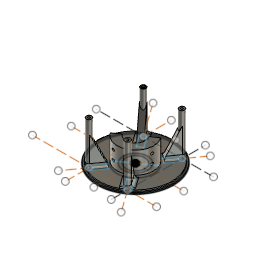
sphere_PS2 v9 (Autodesk Fusion 360 design; units mm, degrees)
Autodesk Fusion 360 part; units mm, degrees
sketch "Skizze1" plane through (0, 0, 0) normal (0, 0, 1) x (1, 0, 0)
  circle A0 centre (0, 0) radius 62.5
  circle A1 centre (0, 0) radius 59.85
  circle A2 centre (0, 0) radius 20
  circle A3 centre (0, 0) radius 15.65
  circle A4 centre (0, 0) radius 6.2
  arc A5 (-24.4487, -17.3857) -> (24.4487, 17.3857) centre (0, 0) ccw
  circle A6 centre (0, 0) radius 2
  line L0 (0, -68.8884) -> (0, 67.0107) construction
  line L1 (80, -45) -> (-125.6154, -45) construction
  line L2 (84.256, 45) -> (-110, 45) construction
  line L3 (32, -72.1137) -> (32, 83.7416) construction
  line L4 (-32, -84.1555) -> (-32, 91.3107) construction
  line L5 (58.3516, -82.0569) -> (-71.7084, 100.84) construction
  line L6 (51.4969, 72.4176) -> (-53.0644, -74.6218) construction
  line L7 (28.3327, -47.6079) -> (15.5832, -29.6788)
  line L8 (35.6673, -42.3921) -> (22.9178, -24.4631)
  line L9 (-28.3327, -47.6079) -> (-15.5832, -29.6788)
  line L10 (-35.6673, -42.3921) -> (-22.9178, -24.4631)
  line L11 (-35.6673, 42.3921) -> (-22.9178, 24.4631)
  line L12 (-28.3327, 47.6079) -> (-15.5832, 29.6788)
  line L13 (28.3327, 47.6079) -> (15.5832, 29.6788)
  line L14 (35.6673, 42.3921) -> (22.9178, 24.4631)
  line L15 (22.9178, -24.4631) -> (15.5832, -29.6788)
  arc A7 (28.3327, -47.6079) -> (35.6673, -42.3921) centre (32, -45) ccw
  line L16 (-15.5832, -29.6788) -> (-22.9178, -24.4631)
  arc A8 (-35.6673, -42.3921) -> (-28.3327, -47.6079) centre (-32, -45) ccw
  line L17 (-15.5832, 29.6788) -> (-22.9178, 24.4631)
  arc A9 (-28.3327, 47.6079) -> (-35.6673, 42.3921) centre (-32, 45) ccw
  line L18 (22.9178, 24.4631) -> (15.5832, 29.6788)
  arc A10 (35.6673, 42.3921) -> (28.3327, 47.6079) centre (32, 45) ccw
  circle A11 centre (32, 45) radius 4.5
  circle A12 centre (-32, 45) radius 4.5
  circle A13 centre (-32, -45) radius 4.5
  circle A14 centre (32, -45) radius 4.5
  line L19 (24.4487, 17.3857) -> (-24.4487, -17.3857)
  line L20 (80, 0) -> (-106.3472, 0) construction
  circle A15 centre (-32, 45) radius 3
  dimension "d1" = 125
  dimension "d2" = 119.7
  dimension "d3" = 40
  dimension "d4" = 31.3
  dimension "d5" = 12.4
  dimension "d6" = 30
  dimension "d15" = 4
  dimension "d54" = 45
  dimension "d55" = 45
  dimension "d56" = 32
  dimension "d57" = 32
  dimension "d66" = 9
  dimension "d67" = 9
  dimension "d68" = 9
  dimension "d69" = 9
  dimension "d100" = 6
  constraint coincident A0.centre A1.centre
  constraint concentric A0 A1
  constraint concentric A3 A6
  constraint vertical L0
  constraint horizontal L2
  constraint vertical L3
  constraint perpendicular L1 L4
  constraint coincident A0.centre L6
  constraint coincident A0.centre L5
  constraint parallel L6 L14
  constraint parallel L6 L13
  constraint parallel L5 L12
  constraint parallel L5 L11
  constraint parallel L6 L10
  constraint parallel L6 L9
  constraint parallel L5 L7
  constraint parallel L5 L8
  constraint perpendicular L5 L15
  constraint coincident L8 L15.start
  constraint coincident L8.end L15.start
  constraint coincident L7 L15.end
  constraint coincident L7.end L15
  constraint coincident L3 A7.centre
  constraint coincident L1 A7.centre
  constraint perpendicular L6 L16
  constraint coincident L10 L16.end
  constraint coincident L9 L16.start
  constraint coincident L9.end L16
  constraint coincident L10.end L16
  constraint coincident L1 A8.centre
  constraint coincident L6 A8.centre
  constraint perpendicular L5 L17
  constraint coincident L11.end L17
  constraint coincident L12 L17.start
  constraint coincident L11 L17.end
  constraint coincident L12.end L17
  constraint coincident L5 A9.centre
  constraint coincident L2 A9.centre
  constraint perpendicular L6 L18
  constraint coincident L13 L18.end
  constraint coincident L14 L18.start
  constraint coincident L14.end L18
  constraint coincident L13.end L18
  constraint coincident L6 A10.centre
  constraint coincident L2 A10.centre
  constraint concentric A10 A11
  constraint concentric A9 A12
  constraint concentric A8 A13
  constraint concentric A7 A14
  constraint coincident A0.centre L19
  constraint horizontal L20
  constraint perpendicular L5 L19
  constraint coincident A5.end L19
  constraint coincident A5.start L19
  constraint coincident A5 L19.end
  constraint coincident A5 L19.start
  constraint concentric A9 A15
  measures "d1" diameter of A0
  measures "d2" diameter of A1
  measures "d3" diameter of A2
  measures "d4" diameter of A3
  measures "d5" diameter of A4
  measures "d6" radius of A5
  measures "d15" diameter of A6
  measures "d54" distance of A0.centre L2
  measures "d55" distance of A0.centre L1
  measures "d56" distance of A0.centre L4
  measures "d57" distance of A0.centre L3
  measures "d66" diameter of A11
  measures "d67" diameter of A12
  measures "d68" diameter of A13
  measures "d69" diameter of A14
  measures "d100" diameter of A15
extrude "Extrusion1" add sketch "Skizze1" along normal blind 2 contours A0 | A1 | A2 A3 L19 | A2 A5 L19 | A2 A3 L19 | A3 A4 L19 | A3 A4 L19 | A4 A6 L19 | A4 A6 L19 | A7 A14 | L7 L8 L15 A14 | L9 L10 L16 A13 | A8 A13 | L11 L12 L17 A12 | A9 A12 | L13 L14 L18 A11 | A10 A11 | A15
extrude "Extrusion2" add sketch "Skizze1" along normal blind 4 contours A1 | A2 A3 L19 | A2 A5 L19 | A2 A3 L19 | A3 A4 L19 | A3 A4 L19 | A7 A14 | L7 L8 L15 A14 | L9 L10 L16 A13 | A8 A13 | L11 L12 L17 A12 | A9 A12 | L13 L14 L18 A11 | A10 A11 | A15
extrude "Extrusion3" add sketch "Skizze1" along normal blind 9 contours A2 A3 L19 | A2 A3 L19
extrude "Extrusion4" add sketch "Skizze1" along normal blind 40 contours A2 A3 L19 | A2 A5 L19 picked at (-14.4863, -11.5112)
extrude "Extrusion10" add sketch "Skizze1" along normal blind 50 contours L7 L8 L15 A14 | L9 L10 L16 A13 | L11 L12 L17 A12 | L13 L14 L18 A11
ref_plane "Arbeitsebene3" through (0, 0, 0) normal (0.814955, -0.579524, 0) x (0.579524, 0.814955, 0)
sketch "Skizze4" plane through (0, 0, 0) normal (0.814955, -0.579524, 0) x (0.579524, 0.814955, 0)
  line L0 (55, 50) -> (33, 50)
  line L1 (-33, 50) -> (-55, 50)
  line L2 (55, 50) -> (33, 4)
  line L3 (73.2312, 4) -> (-81.5781, 4) construction
  line L4 (33, 27.5575) -> (33, -13.6721) construction
  line L5 (-33, 28.7468) -> (-33, -25) construction
  line L6 (55, 50) -> (55, -48.5325) construction
  line L7 (-55, 50) -> (-55, -41.8091) construction
  line L8 (-55, 50) -> (-33, 4)
  line L9 (-33, 4) -> (-33, 50)
  line L10 (33, 4) -> (33, 50)
  point P0 (33, 4)
  point P1 (-33, 4)
  dimension "d72" = 50
  dimension "d73" = 50
  dimension "d75" = 4
  dimension "d76" = 33
  dimension "d77" = 33
  dimension "d78" = 55
  dimension "d79" = 55
  constraint horizontal L0
  constraint horizontal L1
  constraint horizontal L3
  constraint perpendicular L3 L4
  constraint vertical L5
  constraint coincident L4 P0
  constraint coincident L3 P0
  constraint coincident L5 P1
  constraint coincident L3 P1
  constraint coincident L2 P0
  constraint vertical L6
  constraint vertical L7
  constraint coincident L0 L2.start
  constraint coincident L1 L7.start
  constraint coincident L1.end L7
  constraint coincident L0.start L6
  constraint coincident L2 L0.start
  constraint coincident P0 L2.end
  constraint coincident L0.start L2.start
  constraint coincident L1.end L7.start
  constraint coincident P1 L8.end
  constraint coincident L1 L9.end
  constraint perpendicular L1 L9
  constraint coincident L0 L10.end
  constraint perpendicular L0 L10
  constraint coincident L0.end L10
  constraint coincident L1.start L5
  measures "d72" distance of L1 origin
  measures "d73" distance of L0 origin
  measures "d75" distance of L3 origin
  measures "d76" distance of L4 origin
  measures "d77" distance of origin L5
  measures "d78" distance of origin L7
  measures "d79" distance of L6 origin
extrude "Extrusion11" cut sketch "Skizze4" along normal mid plane 20
ref_plane "Arbeitsebene4" through (0, 0, 0) normal (-0.814955, -0.579524, 0) x (0.579524, -0.814955, 0)
sketch "Skizze5" plane through (0, 0, 0) normal (-0.814955, -0.579524, 0) x (0.579524, -0.814955, 0)
  line L0 (-55, 50) -> (-33, 50)
  line L1 (4.8827, 50) -> (55, 50)
  line L2 (-55, 70) -> (-55, -33.6954) construction
  line L3 (55, 69.2155) -> (55, -50) construction
  line L4 (-103.884, 4) -> (120, 4) construction
  line L5 (-33, 50) -> (-33, 4)
  line L6 (33, 50) -> (33, 4)
  line L7 (-55, 50) -> (-33, 4)
  line L8 (55, 50) -> (33, 4)
  dimension "d87" = 50
  dimension "d88" = 50
  dimension "d89" = 55
  dimension "d90" = 55
  dimension "d91" = 4
  dimension "d94" = 22
  dimension "d95" = 22
  constraint horizontal L0
  constraint horizontal L1
  constraint vertical L2
  constraint vertical L3
  constraint horizontal L4
  constraint vertical L5
  constraint perpendicular L4 L6
  constraint coincident L1 L6.start
  constraint coincident L0.end L5
  constraint coincident L0 L5.start
  constraint coincident L4 L5.end
  constraint coincident L4 L6.end
  constraint coincident L1.end L3
  constraint coincident L0.start L2
  constraint coincident L5.end L7.end
  constraint coincident L0.start L7.start
  constraint coincident L6.end L8.end
  constraint coincident L1.end L8.start
  measures "d87" distance of L1 origin
  measures "d88" distance of L0 origin
  measures "d89" distance of origin L2
  measures "d90" distance of origin L3
  measures "d91" distance of origin L4
  measures "d94" distance of L2 L5
  measures "d95" distance of L3 L6
extrude "Extrusion12" cut sketch "Skizze5" along normal mid plane 20
extrude "Extrusion13" add sketch "Skizze1" along normal blind 72 contours A7 A14 | A8 A13 | A10 A11 | A15
extrude "Extrusion14" add sketch "Skizze1" along normal blind 71 contours A9 A12
fillet "Abrundung3" radius 5 3 edges at (-29.2925, 33.4276, 4) (-34.6079, 48.6673, 4) (-21.9579, 38.6433, 4)
fillet "Abrundung4" radius 5 3 edges at (-21.9579, -38.6433, 4) (-34.6079, -48.6673, 4) (-29.2925, -33.4276, 4)
fillet "Abrundung5" radius 5 3 edges at (29.2925, -33.4276, 4) (34.6079, -48.6673, 4) (21.9579, -38.6433, 4)
fillet "Abrundung6" radius 5 3 edges at (21.9579, 38.6433, 4) (34.6079, 48.6673, 4) (29.2925, 33.4276, 4)
ref_plane "Arbeitsebene5" through (-16.2833, -16.4875, 22) normal (-0.579524, 0.814955, 0) x (-0.814955, -0.579524, 0)
sketch "Skizze2" plane through (2.3181, -3.2598, 0) normal (-0.579524, 0.814955, 0) x (0.814955, 0.579524, 0)
  line L0 (23, -47.583) -> (23, 16) construction
  line L1 (-23, -47) -> (-23, 14.5084) construction
  line L2 (39.9606, -30) -> (-42.0458, -30) construction
  line L3 (40.0778, -15) -> (-41.9288, -15) construction
  line L4 (24.6743, -32.9) -> (26.3486, -30)
  line L5 (26.3486, -30) -> (24.6743, -27.1)
  line L6 (24.6743, -27.1) -> (21.3257, -27.1)
  line L7 (21.3257, -27.1) -> (19.6514, -30)
  line L8 (19.6514, -30) -> (21.3257, -32.9)
  line L9 (21.3257, -32.9) -> (24.6743, -32.9)
  line L10 (24.6743, -17.9) -> (26.3486, -15)
  line L11 (26.3486, -15) -> (24.6743, -12.1)
  line L12 (24.6743, -12.1) -> (21.3257, -12.1)
  line L13 (21.3257, -12.1) -> (19.6514, -15)
  line L14 (19.6514, -15) -> (21.3257, -17.9)
  line L15 (21.3257, -17.9) -> (24.6743, -17.9)
  line L16 (-21.3257, -32.9) -> (-19.6514, -30)
  line L17 (-19.6514, -30) -> (-21.3257, -27.1)
  line L18 (-21.3257, -27.1) -> (-24.6743, -27.1)
  line L19 (-24.6743, -27.1) -> (-26.3486, -30)
  line L20 (-26.3486, -30) -> (-24.6743, -32.9)
  line L21 (-24.6743, -32.9) -> (-21.3257, -32.9)
  line L22 (-21.3257, -17.9) -> (-19.6514, -15)
  line L23 (-19.6514, -15) -> (-21.3257, -12.1)
  line L24 (-21.3257, -12.1) -> (-24.6743, -12.1)
  line L25 (-24.6743, -12.1) -> (-26.3486, -15)
  line L26 (-26.3486, -15) -> (-24.6743, -17.9)
  line L27 (-24.6743, -17.9) -> (-21.3257, -17.9)
  line L28 (26.3486, -32.9) -> (19.6514, -32.9)
  line L29 (19.6514, -32.9) -> (19.6514, -30)
  line L30 (19.6514, -30) -> (26.3486, -30)
  line L31 (26.3486, -30) -> (26.3486, -32.9)
  line L32 (-19.6514, -32.9) -> (-26.3486, -32.9)
  line L33 (-26.3486, -32.9) -> (-26.3486, -30)
  line L34 (-26.3486, -30) -> (-19.6514, -30)
  line L35 (-19.6514, -30) -> (-19.6514, -32.9)
  line L36 (-19.6514, -17.9) -> (-26.3486, -17.9)
  line L37 (-26.3486, -17.9) -> (-26.3486, -15)
  line L38 (-26.3486, -15) -> (-19.6514, -15)
  line L39 (-19.6514, -15) -> (-19.6514, -17.9)
  line L40 (26.3486, -17.9) -> (19.6514, -17.9)
  line L41 (19.6514, -17.9) -> (19.6514, -15)
  line L42 (19.6514, -15) -> (26.3486, -15)
  line L43 (26.3486, -15) -> (26.3486, -17.9)
  circle A0 centre (23, -30) radius 1.75
  circle A1 centre (23, -15) radius 1.75
  circle A2 centre (-23, -30) radius 1.75
  circle A3 centre (-23, -15) radius 1.75
  line L44 (-15.65, -9) -> (-20, -9)
  line L45 (-20, -9) -> (-20, -4)
  line L46 (-20, -4) -> (-30, -4)
  line L47 (-30, -4) -> (-30, -40)
  line L48 (-30, -40) -> (-15.65, -40)
  line L49 (-15.65, -40) -> (-15.65, -9)
  line L50 (67, 0) -> (-48, 0) construction
  line L51 (83.9354, 0) -> (-86.4902, 0)
  line L52 (-15.713, 0) -> (74.6088, 0)
  point P0 (23, -30)
  point P1 (23, -15)
  point P2 (-23, -15)
  point P3 (-23, -30)
  point P4 (23, -30)
  point P5 (23, -15)
  point P6 (-23, -30)
  point P7 (-23, -15)
  dimension "d24" = 23
  dimension "d25" = 23
  dimension "d26" = 30
  dimension "d27" = 15
  dimension "d28" = 5.8
  dimension "d29" = 5.8
  dimension "d30" = 5.8
  dimension "d31" = 5.8
  dimension "d32" = 3.5
  dimension "d33" = 3.5
  dimension "d34" = 3.5
  dimension "d35" = 3.5
  constraint vertical L0
  constraint vertical L1
  constraint coincident L2 P4
  constraint coincident L0 P4
  constraint coincident L3 P5
  constraint coincident L0 P5
  constraint coincident L1 P7
  constraint coincident L3 P7
  constraint coincident L1 P6
  constraint coincident L2 P6
  constraint coincident P4 P0
  constraint coincident P5 P1
  constraint coincident P6 P3
  constraint coincident P7 P2
  constraint horizontal L28
  constraint vertical L29
  constraint horizontal L30
  constraint vertical L31
  constraint coincident P4 L30
  constraint coincident L7.end L8.start
  constraint coincident L4.end L5.start
  constraint coincident L8.end L28
  constraint horizontal L32
  constraint vertical L33
  constraint horizontal L34
  constraint vertical L35
  constraint coincident P6 L34
  constraint coincident L19.end L20.start
  constraint coincident L16.end L17.start
  constraint coincident L16.start L32
  constraint horizontal L36
  constraint vertical L37
  constraint horizontal L38
  constraint vertical L39
  constraint coincident P7 L38
  constraint coincident L25.end L26.start
  constraint coincident L26.end L36
  constraint coincident L22.end L23.start
  constraint horizontal L40
  constraint vertical L41
  constraint horizontal L42
  constraint vertical L43
  constraint coincident P5 L42
  constraint coincident L13.end L14.start
  constraint coincident L10.end L11.start
  constraint coincident L14.end L40
  constraint horizontal L50
  constraint coincident L50 origin
  constraint parallel L2 L51
  constraint parallel L3 L52
  measures "d24" distance of L0 origin
  measures "d25" distance of L1 origin
  measures "d26" distance of origin L2
  measures "d27" distance of origin L3
  measures "d28" distance of L6 L9
  measures "d29" distance of L12 L15
  measures "d30" distance of L18 L21
  measures "d31" distance of L24 L27
  measures "d32" diameter of A3
  measures "d33" diameter of A2
  measures "d34" diameter of A0
  measures "d35" diameter of A1
extrude "Extrusion6" cut sketch "Skizze2" along normal mid plane 80 contours L30 A0 | L30 A0 | L42 A1 | L42 A1 | L34 A2 | L34 A2 | L38 A3 | L38 A3
extrude "Extrusion7" cut sketch "Skizze2" along normal mid plane 2.8 contours L4 L8 L9 L28 L30 A0 | L4 L28 L31 | L5 L6 L7 L30 A0 | L8 L28 L29 | L10 L14 L15 L40 L42 A1 | L10 L40 L43 | L11 L12 L13 L42 A1 | L14 L40 L41 | L16 L20 L21 L32 L34 A2 | L16 L32 L35 | L17 L18 L19 L34 A2 | L20 L32 L33 | L22 L26 L27 L36 L38 A3 | L22 L36 L39 | L23 L24 L25 L38 A3 | L26 L36 L37
ref_plane "Arbeitsebene2" through (-32, -45, 66) normal (0, 0, 1) x (1, 0, 0)
sketch "Skizze3" plane through (0, 0, 66) normal (0, 0, 1) x (1, 0, 0)
  line L0 (47.2936, -66.5067) -> (-50.249, 70.6626) construction
  line L1 (-42.6718, -60.0072) -> (38.3749, 53.9647) construction
  line L2 (-31.9062, -41.6527) -> (-34.852, -43.2451)
  line L3 (-34.852, -43.2451) -> (-34.9457, -46.5925)
  line L4 (-34.9457, -46.5925) -> (-32.0938, -48.3473)
  line L5 (-32.0938, -48.3473) -> (-29.148, -46.7549)
  line L6 (-29.148, -46.7549) -> (-29.0543, -43.4075)
  line L7 (-29.0543, -43.4075) -> (-31.9062, -41.6527)
  line L8 (-28.9183, 43.6898) -> (-29.3245, 47.0137)
  line L9 (-29.3245, 47.0137) -> (-32.4061, 48.3239)
  line L10 (-32.4061, 48.3239) -> (-35.0817, 46.3102)
  line L11 (-35.0817, 46.3102) -> (-34.6755, 42.9863)
  line L12 (-34.6755, 42.9863) -> (-31.5939, 41.6761)
  line L13 (-31.5939, 41.6761) -> (-28.9183, 43.6898)
  line L14 (31.9063, 41.6527) -> (34.852, 43.2452)
  line L15 (34.852, 43.2452) -> (34.9457, 46.5925)
  line L16 (34.9457, 46.5925) -> (32.0937, 48.3473)
  line L17 (32.0937, 48.3473) -> (29.148, 46.7548)
  line L18 (29.148, 46.7548) -> (29.0543, 43.4075)
  line L19 (29.0543, 43.4075) -> (31.9063, 41.6527)
  line L20 (35.0817, -46.3102) -> (34.6755, -42.9863)
  line L21 (34.6755, -42.9863) -> (31.5939, -41.6761)
  line L22 (31.5939, -41.6761) -> (28.9183, -43.6898)
  line L23 (28.9183, -43.6898) -> (29.3245, -47.0137)
  line L24 (29.3245, -47.0137) -> (32.4061, -48.3239)
  line L25 (32.4061, -48.3239) -> (35.0817, -46.3102)
  circle A0 centre (-32, 45) radius 1.75
  circle A1 centre (-32, -45) radius 1.75
  circle A2 centre (32, -45) radius 1.75
  circle A3 centre (32, 45) radius 1.75
  line L26 (-32, -63.1927) -> (-32, 71.2003) construction
  line L27 (-86.7098, 45) -> (100, 45) construction
  line L28 (-83.1793, -45) -> (68.6306, -45) construction
  line L29 (32, -70) -> (32, 90) construction
  point P0 (-32, -45)
  point P1 (-32, 45)
  point P2 (32, 45)
  point P3 (32, -45)
  point P4 (-32, -45)
  point P5 (-32, 45)
  point P6 (32, 45)
  point P7 (32, -45)
  point P8 (-32, 45)
  point P9 (102.7985, 45)
  point P10 (-3.6645, -45)
  point P11 (-32, -45)
  point P12 (32, 45)
  point P13 (32, -45)
  dimension "d42" = 5.8
  dimension "d43" = 5.8
  dimension "d44" = 5.8
  dimension "d45" = 5.8
  dimension "d46" = 3.5
  dimension "d47" = 3.5
  dimension "d48" = 3.5
  dimension "d49" = 3.5
  dimension "d113" = 32
  dimension "d114" = 45
  dimension "d115" = 45
  dimension "d116" = 32
  constraint coincident L0 origin
  constraint coincident origin L1
  constraint coincident L1 P11
  constraint coincident L0 P8
  constraint coincident L1 P12
  constraint coincident L0 P13
  constraint coincident P11 P4
  constraint coincident P8 P5
  constraint coincident P12 P6
  constraint coincident P13 P7
  constraint vertical L26
  constraint horizontal L27
  constraint horizontal L28
  constraint coincident L27 P8
  constraint coincident L26 P8
  constraint coincident L27 P9
  constraint coincident L28 P10
  constraint coincident L28 P11
  constraint coincident L26 P11
  constraint perpendicular L28 L29
  constraint coincident L27 P12
  constraint coincident L28 P13
  measures "d42" distance of L4 L7
  measures "d43" distance of L16 L19
  measures "d44" distance of L10 L13
  measures "d45" distance of L22 L25
  measures "d46" diameter of A3
  measures "d47" diameter of A2
  measures "d48" diameter of A1
  measures "d49" diameter of A0
  measures "d113" distance of origin L26
  measures "d114" distance of origin L28
  measures "d115" distance of origin L27
  measures "d116" distance of origin L29
extrude "Extrusion15" cut sketch "Skizze3" along normal mid plane 20 contours A0 | A1 | A2 | A3
extrude "Extrusion16" cut sketch "Skizze3" along normal blind 2.8
sketch "Skizze7" plane through (0, 0, 0) normal (-0.579524, 0.814955, 0) x (-0.814955, -0.579524, 0)
  circle A0 centre (23, 15) radius 1.75
  circle A1 centre (23, 30) radius 1.75
  line L0 (15.65, 9) -> (20, 9)
  line L1 (20, 9) -> (20, 4)
  line L2 (20, 4) -> (30, 4)
  line L3 (30, 4) -> (30, 40)
  line L4 (30, 40) -> (15.65, 40)
  line L5 (15.65, 40) -> (15.65, 9)
  line L6 (0, 29.5362) -> (0, -19.182) construction
  line L7 (-27.8769, 9.5) -> (35.5762, 9.5) construction
  circle A2 centre (0, 9.5) radius 4.5
  dimension "d125" = 9.5
  dimension "d126" = 9
  constraint vertical L6
  constraint coincident L6 origin
  constraint perpendicular L3 L7
  constraint coincident L7 A2.centre
  constraint coincident L6 A2.centre
  measures "d125" distance of origin L7
  measures "d126" diameter of A2
extrude "Extrusion18" cut sketch "Skizze7" along normal blind 30 contours A2
